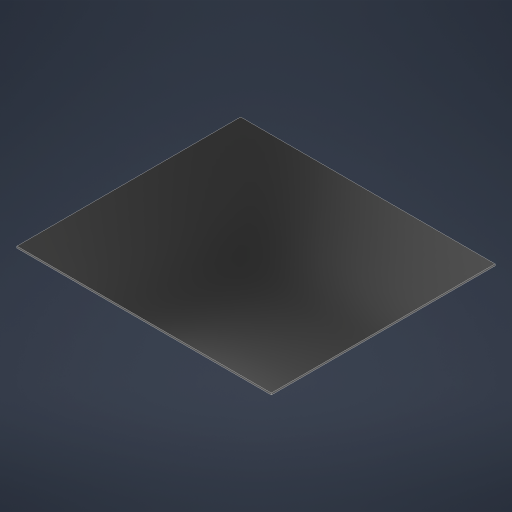
# Autodesk Inventor part: Piano cottura
Saved by Autodesk Inventor 2024.2 (Build 282272000, 272)
## iProperties
Created: 2025-08-23
Part Number: Piano cottura
Material: Generic
Document SubType Name: Modeling
Designer: Luca
Density: 1 g/cm^3
Appearance: Glazed - Black
Author: Luca
Autodesk Inventor part; units mm, degrees
ref_plane "YZ Plane" through (0, 0, 0) normal (1, 0, 0) x (0, 1, 0)
ref_plane "XZ Plane" through (0, 0, 0) normal (0, 1, 0) x (-1, 0, 0)
ref_plane "XY Plane" through (0, 0, 0) normal (0, 0, 1) x (1, 0, 0)
sketch "Sketch1" plane through (0, 0, 0) normal (0, 1, 0) x (-1, 0, 0)
  line L0 (290, 255) -> (-290, 255)
  line L1 (-290, 255) -> (-290, -255)
  line L2 (-290, -255) -> (290, -255)
  line L3 (290, -255) -> (290, 255)
  line L4 (290, 255) -> (-290, -255) construction
  line L5 (-290, 255) -> (290, -255) construction
  point P0 (0, 0)
  dimension "d0" = 580
  dimension "d1" = 510
  constraints: 12 end point, 2 midpoint, 2 parallel, 1 horizontal, 1 perpendicular
  measures "d0" distance of L2.end L1.end
  measures "d1" distance of L1.end L0.end
extrude "Extrusion1" add sketch "Sketch1" against normal blind 4
body "Solid1"
